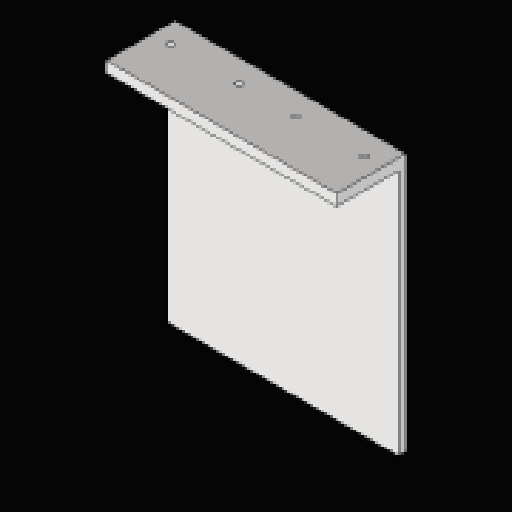
# Autodesk Inventor part: Frame
Saved by Autodesk Inventor 2023.2 (Build 272271030, 271C)
## iProperties
Created: 2023-11-06
Part Number: Frame
Material: Generic
Document SubType Name: Modeling
Designer: robpl
Density: 1 g/cm^3
Appearance: Default
Author: robpl
Autodesk Inventor part; units mm, degrees
ref_plane "YZ Plane" through (0, 0, 0) normal (1, 0, 0) x (0, 1, 0)
ref_plane "XZ Plane" through (0, 0, 0) normal (0, 1, 0) x (-1, 0, 0)
ref_plane "XY Plane" through (0, 0, 0) normal (0, 0, 1) x (1, 0, 0)
sketch "Sketch1" plane through (0, 0, 0) normal (0, 0, 1) x (1, 0, 0)
  line L0 (0, 0) -> (93.4, 0)
  line L1 (93.4, 0) -> (93.4, 100)
  line L2 (93.4, 100) -> (0, 100)
  line L3 (0, 100) -> (0, 0)
  dimension "d0" = 93.4
  dimension "d1" = 100
  constraints: 8 end point, 2 parallel, 1 horizontal, 1 perpendicular
  measures "d0" distance of L2.end L1.end
  measures "d1" distance of L1.end L0.end
extrude "Extrusion1" add sketch "Sketch1" along normal blind 3
sketch "Sketch2" plane through (0, 100, 0) normal (0, 1, 0) x (1, 0, 0)
  line L0 (0, 0) -> (0, -3) projected
  line L1 (0, 0) -> (93.4, 0)
  line L2 (93.4, 0) -> (93.4, -28)
  line L3 (93.4, -28) -> (0, -28)
  line L4 (0, -28) -> (0, 0)
  line L5 (93.4, 0) -> (0, 0) projected
  line L6 (0, 0) -> (0, -3) projected
  line L7 (93.4, -3) -> (0, -3) projected
  line L8 (93.4, 0) -> (93.4, -3) projected
  line L9 (93.4, -3) -> (0, -3) projected
  line L10 (83.6, -20.35) -> (60.6, -20.35)
  line L11 (60.6, -20.35) -> (60.6, -7.65)
  line L12 (60.6, -7.65) -> (83.6, -7.65)
  line L13 (83.6, -7.65) -> (83.6, -20.35)
  line L14 (32.8, -7.65) -> (9.8, -7.65)
  line L15 (9.8, -7.65) -> (9.8, -20.35)
  line L16 (9.8, -20.35) -> (32.8, -20.35)
  line L17 (32.8, -20.35) -> (32.8, -7.65)
  arc A0 (86.9526, -8.8) -> (86.9526, -9.9) centre (86, -9.35) ccw projected
  arc A1 (57.2474, -9.9) -> (57.2474, -8.8) centre (58.2, -9.35) ccw projected
  arc A2 (36.1526, -8.8) -> (36.1526, -9.9) centre (35.2, -9.35) ccw projected
  arc A3 (6.4474, -9.9) -> (6.4474, -8.8) centre (7.4, -9.35) ccw projected
  circle A4 centre (7.4, -14) radius 1.25
  circle A5 centre (35.2, -14) radius 1.25
  circle A6 centre (58.2, -14) radius 1.25
  circle A7 centre (86, -14) radius 1.25
  point P0 (9.8, -3)
  point P1 (32.8, -3)
  point P2 (60.6, -3)
  point P3 (83.6, -3)
  point P4 (32.8, -14)
  dimension "d4" = 3
  dimension "d6" = 9.8
  dimension "d7" = 7.65
  dimension "d8" = 23
  dimension "d9" = 9.8
  dimension "d13" = 12.7
  dimension "d14" = 28
  dimension "d15" = 7.65
  dimension "d16" = 2.5
  constraints: 24 end point, 6 parallel, 5 horizontal alignment, 4 centre point, 4 vertical alignment, 3 equal radius, 3 horizontal, 3 perpendicular, 2 equal length, 1 midpoint
  measures "d4" distance between parallel lines of L1 L7
  measures "d6" distance between parallel lines of L2 L13
  measures "d7" distance between parallel lines of L3 L10
  measures "d8" distance of L10.start L10.end
  measures "d9" distance between parallel lines of L4 L15
  measures "d13" distance of L12.end L10.start
  measures "d14" distance between parallel lines of L3 L1
  measures "d15" distance between parallel lines of L1 L12
  measures "d16" diameter of A4
extrude "Extrusion2" add sketch "Sketch2" along normal blind 4.5
sketch "Sketch3" plane through (0, 104.5, 0) normal (0, 1, 0) x (1, 0, 0)
  line L0 (93.4, -28) -> (93.4, 0) projected
  line L1 (93.4, 0) -> (0, 0) projected
  line L2 (0, 0) -> (0, -28) projected
  line L3 (0, -28) -> (93.4, -28) projected
  circle A0 centre (86, -14) radius 1.25 projected
  circle A1 centre (7.4, -14) radius 1.25 projected
  circle A2 centre (35.2, -14) radius 1.25 projected
  circle A3 centre (58.2, -14) radius 1.25 projected
  line L4 (32.8, -7.65) -> (32.8, -20.35) projected
  line L5 (32.8, -20.35) -> (9.8, -20.35) projected
  line L6 (9.8, -20.35) -> (9.8, -7.65) projected
  line L7 (9.8, -7.65) -> (32.8, -7.65) projected
  line L8 (83.6, -20.35) -> (60.6, -20.35) projected
  line L9 (60.6, -20.35) -> (60.6, -7.65) projected
  line L10 (60.6, -7.65) -> (83.6, -7.65) projected
  line L11 (83.6, -7.65) -> (83.6, -20.35) projected
  line L12 (88.4, -24.5) -> (5, -24.5)
  line L13 (5, -24.5) -> (5, -3.5)
  line L14 (5, -3.5) -> (88.4, -3.5)
  line L15 (88.4, -3.5) -> (88.4, -24.5)
  point P0 (88.4, -14)
  point P1 (93.4, -14)
  dimension "d17" = 5
  dimension "d18" = 5
  dimension "d19" = 21
  constraints: 8 end point, 2 midpoint, 2 parallel, 1 horizontal, 1 horizontal alignment, 1 perpendicular
  measures "d17" distance between parallel lines of L2 L13
  measures "d18" distance between parallel lines of L0 L15
  measures "d19" distance between parallel lines of L14 L12
equation "\"d7\" = d15"
equation "\"d9\" = d6"
equation "\"d18\" = d17"
body "Solid1"
